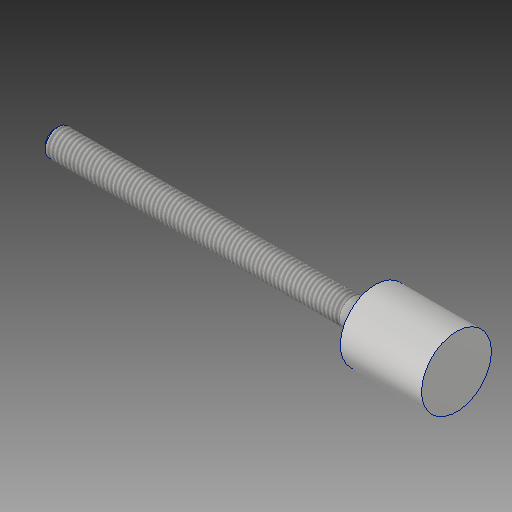
# Autodesk Inventor part: 螺桿
Saved by Autodesk Inventor 2017 (Build 210142000, 142)
## iProperties
Part Number: 螺桿
Material: 鋁合金 6061
Document SubType Name: Modeling
Designer: user
Density: 2.7 g/cm^3
Appearance: 鋁 - 平面
Author: user
Autodesk Inventor part; units mm, degrees
ref_plane "YZ Plane" through (0, 0, 0) normal (1, 0, 0) x (0, 1, 0)
ref_plane "XZ Plane" through (0, 0, 0) normal (0, 1, 0) x (-1, 0, 0)
ref_plane "XY Plane" through (0, 0, 0) normal (0, 0, 1) x (1, 0, 0)
sketch "草圖1" plane through (0, 0, 0) normal (0, 0, 1) x (1, 0, 0)
  line L0 (0, 0) -> (0, 12.55)
  line L1 (0, 12.55) -> (-29.22, 12.55)
  line L2 (-29.22, 12.55) -> (-29.22, 4.75)
  line L3 (-29.22, 4.75) -> (-144.22, 4.75)
  line L4 (-144.22, 4.75) -> (-144.22, 0)
  line L5 (-144.22, 0) -> (0, 0)
  dimension "d0" = 29.22
  dimension "d1" = 12.55
  dimension "d2" = 115
  dimension "d3" = 4.75
  constraints: 12 end point, 3 perpendicular, 2 horizontal, 1 horizontal alignment, 1 vertical
  measures "d0" distance of L0.end L1.end
  measures "d1" distance of L0.start L0.end
  measures "d2" distance of L2.end L3.end
  measures "d3" distance of L3.end L4.end
revolve "迴轉1" add sketch "草圖1" angle 360 about axis through (-144.22, 0, 0) along (1, 0, 0)
chamfer "倒角1" distance 1 angle 45 1 edges at (-144.22, -4.75, 0)
thread "螺紋1" size "M10x1.5" class "6g" standard "ANSI Metric M Profile" length 105.9
sketch "草圖2" plane through (-144.22, 0, 0) normal (-1, 0, 0) x (0, 0, 1)
  circle A0 centre (0, 0) radius 2
  dimension "d10" = 4
  constraints: 1 centre point, 1 coincident
  measures "d10" diameter of A0
extrude "擠出1" cut sketch "草圖2" against normal blind 3.8
